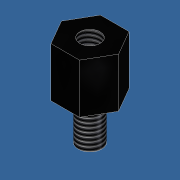
# Autodesk Inventor part: Entretoise_M3x6
Saved by Autodesk Inventor 2015 SP2 (Build 190223200, 223)
## iProperties
Created: 2017-10-31
Part Number: Entretoise_M3x6
Project: Nom Projet
Material: .
Description: Nom pièce
Document SubType Name: Modeling
Designer: Benoit.CURCHOD2
Authority: brut Ø
Density: 0.001 g/cm^3
Appearance: Noir
Material number: ---
Author: Benoit.CURCHOD2
Autodesk Inventor part; units mm, degrees
ref_plane "Plan YZ" through (0, 0, 0) normal (1, 0, 0) x (0, 1, 0)
ref_plane "Plan XZ" through (0, 0, 0) normal (0, 1, 0) x (-1, 0, 0)
ref_plane "Plan XY" through (0, 0, 0) normal (0, 0, 1) x (1, 0, 0)
sketch "Esquisse1" plane through (0, 0, 0) normal (0, 0, 1) x (1, 0, 0)
  circle A0 centre (0, 0) radius 1.425
  dimension "d0" = 2.85
  constraints: 1 centre point, 1 coincident
  measures "d0" diameter of A0
extrude "Extrusion1" add sketch "Esquisse1" along normal blind 5
sketch "Esquisse6" plane through (0, 0, 5) normal (0, 0, 1) x (1, 0, 0)
  line L0 (-4.8497, 0) -> (4.8497, 0) construction
  line L1 (0, -4.2) -> (0, 4.2) construction
  line L2 (-1.7321, -3) -> (-3.4641, 0)
  line L3 (-3.4641, 0) -> (-1.7321, 3)
  line L4 (-1.7321, 3) -> (0, 3)
  line L5 (-1.7321, -3) -> (0, -3)
  line L6 (1.7321, -3) -> (3.4641, 0)
  line L7 (3.4641, 0) -> (1.7321, 3)
  line L8 (1.7321, 3) -> (0, 3)
  line L9 (1.7321, -3) -> (0, -3)
  point P0 (0, 0)
  dimension "d4" = 6
  dimension "d8" = 120
  dimension "d10" = 6
  constraints: 16 end point, 3 point on line, 3 symmetric about line, 2 perpendicular, 2 other
  measures "d4" distance between parallel lines of L5 L4
  measures "d8" angle of L2 L3
  measures "d10" distance between parallel lines of L6 L3
extrude "Extrusion2" add sketch "Esquisse6" along normal blind 6
sketch "Esquisse7" plane through (0, 0, 11) normal (0, 0, 1) x (1, 0, 0)
  circle A0 centre (0, 0) radius 1.425 projected
hole "Perçage1" at (0, 0, 11) direction (0, 0, -1) diameter 2.459 depth 5 tip angle 118 thread size "M3x0.5" class "6H" standard "ISO M"
thread "Filetage1" size "M3x0.5" class "6g" standard "ISO M" full length
